Autodesk Fusion 360 part; units mm, degrees
(part 8 of 12)
  arc A873 (-163.0531, -58.1721) -> (-160.5131, -58.1721) centre (-161.7831, -58.1721) ccw
  arc A874 (-124.1631, -55.6321) -> (-126.7031, -55.6321) centre (-125.4331, -55.6321) ccw
  arc A875 (-126.7031, -55.6321) -> (-124.1631, -55.6321) centre (-125.4331, -55.6321) ccw
  arc A876 (-126.7031, -55.6321) -> (-124.1631, -55.6321) centre (-125.4331, -55.6321) ccw
  arc A877 (-124.1631, -55.6321) -> (-126.7031, -55.6321) centre (-125.4331, -55.6321) ccw
  arc A878 (-124.1631, -55.6321) -> (-126.7031, -55.6321) centre (-125.4331, -55.6321) ccw
  arc A879 (-126.7031, -55.6321) -> (-124.1631, -55.6321) centre (-125.4331, -55.6321) ccw
  arc A880 (-130.5131, -58.1721) -> (-133.0531, -58.1721) centre (-131.7831, -58.1721) ccw
  arc A881 (-133.0531, -58.1721) -> (-130.5131, -58.1721) centre (-131.7831, -58.1721) ccw
  arc A882 (-133.0531, -58.1721) -> (-130.5131, -58.1721) centre (-131.7831, -58.1721) ccw
  arc A883 (-130.5131, -58.1721) -> (-133.0531, -58.1721) centre (-131.7831, -58.1721) ccw
  arc A884 (-130.5131, -58.1721) -> (-133.0531, -58.1721) centre (-131.7831, -58.1721) ccw
  arc A885 (-133.0531, -58.1721) -> (-130.5131, -58.1721) centre (-131.7831, -58.1721) ccw
  arc A886 (-94.1631, -55.6321) -> (-96.7031, -55.6321) centre (-95.4331, -55.6321) ccw
  arc A887 (-96.7031, -55.6321) -> (-94.1631, -55.6321) centre (-95.4331, -55.6321) ccw
  arc A888 (-96.7031, -55.6321) -> (-94.1631, -55.6321) centre (-95.4331, -55.6321) ccw
  arc A889 (-94.1631, -55.6321) -> (-96.7031, -55.6321) centre (-95.4331, -55.6321) ccw
  arc A890 (-96.7031, -55.6321) -> (-94.1631, -55.6321) centre (-95.4331, -55.6321) ccw
  arc A891 (-94.1631, -55.6321) -> (-96.7031, -55.6321) centre (-95.4331, -55.6321) ccw
  arc A892 (-103.0531, -58.1721) -> (-100.5131, -58.1721) centre (-101.7831, -58.1721) ccw
  arc A893 (-100.5131, -58.1721) -> (-103.0531, -58.1721) centre (-101.7831, -58.1721) ccw
  arc A894 (-103.0531, -58.1721) -> (-100.5131, -58.1721) centre (-101.7831, -58.1721) ccw
  arc A895 (-100.5131, -58.1721) -> (-103.0531, -58.1721) centre (-101.7831, -58.1721) ccw
  arc A896 (-103.0531, -58.1721) -> (-100.5131, -58.1721) centre (-101.7831, -58.1721) ccw
  arc A897 (-100.5131, -58.1721) -> (-103.0531, -58.1721) centre (-101.7831, -58.1721) ccw
  arc A898 (-66.7031, -55.6321) -> (-64.1631, -55.6321) centre (-65.4331, -55.6321) ccw
  arc A899 (-64.1631, -55.6321) -> (-66.7031, -55.6321) centre (-65.4331, -55.6321) ccw
  arc A900 (-64.1631, -55.6321) -> (-66.7031, -55.6321) centre (-65.4331, -55.6321) ccw
  arc A901 (-66.7031, -55.6321) -> (-64.1631, -55.6321) centre (-65.4331, -55.6321) ccw
  arc A902 (-64.1631, -55.6321) -> (-66.7031, -55.6321) centre (-65.4331, -55.6321) ccw
  arc A903 (-66.7031, -55.6321) -> (-64.1631, -55.6321) centre (-65.4331, -55.6321) ccw
  arc A904 (-70.5131, -58.1721) -> (-73.0531, -58.1721) centre (-71.7831, -58.1721) ccw
  arc A905 (-73.0531, -58.1721) -> (-70.5131, -58.1721) centre (-71.7831, -58.1721) ccw
  arc A906 (-73.0531, -58.1721) -> (-70.5131, -58.1721) centre (-71.7831, -58.1721) ccw
  arc A907 (-70.5131, -58.1721) -> (-73.0531, -58.1721) centre (-71.7831, -58.1721) ccw
  arc A908 (-73.0531, -58.1721) -> (-70.5131, -58.1721) centre (-71.7831, -58.1721) ccw
  arc A909 (-70.5131, -58.1721) -> (-73.0531, -58.1721) centre (-71.7831, -58.1721) ccw
  arc A910 (-34.1631, -55.6321) -> (-36.7031, -55.6321) centre (-35.4331, -55.6321) ccw
  arc A911 (-36.7031, -55.6321) -> (-34.1631, -55.6321) centre (-35.4331, -55.6321) ccw
  arc A912 (-34.1631, -55.6321) -> (-36.7031, -55.6321) centre (-35.4331, -55.6321) ccw
  arc A913 (-36.7031, -55.6321) -> (-34.1631, -55.6321) centre (-35.4331, -55.6321) ccw
  arc A914 (-34.1631, -55.6321) -> (-36.7031, -55.6321) centre (-35.4331, -55.6321) ccw
  arc A915 (-36.7031, -55.6321) -> (-34.1631, -55.6321) centre (-35.4331, -55.6321) ccw
  arc A916 (-43.0531, -58.1721) -> (-40.5131, -58.1721) centre (-41.7831, -58.1721) ccw
  arc A917 (-40.5131, -58.1721) -> (-43.0531, -58.1721) centre (-41.7831, -58.1721) ccw
  arc A918 (-40.5131, -58.1721) -> (-43.0531, -58.1721) centre (-41.7831, -58.1721) ccw
  arc A919 (-43.0531, -58.1721) -> (-40.5131, -58.1721) centre (-41.7831, -58.1721) ccw
  arc A920 (-43.0531, -58.1721) -> (-40.5131, -58.1721) centre (-41.7831, -58.1721) ccw
  arc A921 (-40.5131, -58.1721) -> (-43.0531, -58.1721) centre (-41.7831, -58.1721) ccw
  arc A922 (8.763, -56.6421) -> (6.223, -56.6421) centre (7.493, -56.6421) ccw
  arc A923 (6.223, -56.6421) -> (8.763, -56.6421) centre (7.493, -56.6421) ccw
  arc A924 (6.223, -56.6421) -> (8.763, -56.6421) centre (7.493, -56.6421) ccw
  arc A925 (8.763, -56.6421) -> (6.223, -56.6421) centre (7.493, -56.6421) ccw
  arc A926 (6.223, -56.6421) -> (8.763, -56.6421) centre (7.493, -56.6421) ccw
  arc A927 (8.763, -56.6421) -> (6.223, -56.6421) centre (7.493, -56.6421) ccw
  arc A928 (2.413, -59.1821) -> (-0.127, -59.1821) centre (1.143, -59.1821) ccw
  arc A929 (-0.127, -59.1821) -> (2.413, -59.1821) centre (1.143, -59.1821) ccw
  arc A930 (-0.127, -59.1821) -> (2.413, -59.1821) centre (1.143, -59.1821) ccw
  arc A931 (2.413, -59.1821) -> (-0.127, -59.1821) centre (1.143, -59.1821) ccw
  arc A932 (-0.127, -59.1821) -> (2.413, -59.1821) centre (1.143, -59.1821) ccw
  arc A933 (2.413, -59.1821) -> (-0.127, -59.1821) centre (1.143, -59.1821) ccw
  arc A934 (-175.4509, -86.7412) -> (-172.9108, -86.7412) centre (-174.1808, -86.7412) ccw
  arc A935 (-172.9108, -86.7412) -> (-175.4509, -86.7412) centre (-174.1808, -86.7412) ccw
  arc A936 (-175.4509, -86.7412) -> (-172.9108, -86.7412) centre (-174.1808, -86.7412) ccw
  arc A937 (-172.9108, -86.7412) -> (-175.4509, -86.7412) centre (-174.1808, -86.7412) ccw
  arc A938 (-172.9108, -86.7412) -> (-175.4509, -86.7412) centre (-174.1808, -86.7412) ccw
  arc A939 (-175.4509, -86.7412) -> (-172.9108, -86.7412) centre (-174.1808, -86.7412) ccw
  arc A940 (-181.8009, -89.2812) -> (-179.2609, -89.2812) centre (-180.5309, -89.2812) ccw
  arc A941 (-179.2609, -89.2812) -> (-181.8009, -89.2812) centre (-180.5309, -89.2812) ccw
  arc A942 (-181.8009, -89.2812) -> (-179.2609, -89.2812) centre (-180.5309, -89.2812) ccw
  arc A943 (-179.2609, -89.2812) -> (-181.8009, -89.2812) centre (-180.5309, -89.2812) ccw
  arc A944 (-181.8009, -89.2812) -> (-179.2609, -89.2812) centre (-180.5309, -89.2812) ccw
  arc A945 (-179.2609, -89.2812) -> (-181.8009, -89.2812) centre (-180.5309, -89.2812) ccw
  arc A946 (57.6581, -64.0081) -> (55.1181, -64.0081) centre (56.3881, -64.0081) ccw
  arc A947 (55.1181, -64.0081) -> (57.6581, -64.0081) centre (56.3881, -64.0081) ccw
  arc A948 (55.1181, -64.0081) -> (57.6581, -64.0081) centre (56.3881, -64.0081) ccw
  arc A949 (57.6581, -64.0081) -> (55.1181, -64.0081) centre (56.3881, -64.0081) ccw
  arc A950 (55.1181, -64.0081) -> (57.6581, -64.0081) centre (56.3881, -64.0081) ccw
  arc A951 (57.6581, -64.0081) -> (55.1181, -64.0081) centre (56.3881, -64.0081) ccw
  arc A952 (48.7681, -66.5481) -> (51.3081, -66.5481) centre (50.0381, -66.5481) ccw
  arc A953 (51.3081, -66.5481) -> (48.7681, -66.5481) centre (50.0381, -66.5481) ccw
  arc A954 (48.7681, -66.5481) -> (51.3081, -66.5481) centre (50.0381, -66.5481) ccw
  arc A955 (51.3081, -66.5481) -> (48.7681, -66.5481) centre (50.0381, -66.5481) ccw
  arc A956 (51.3081, -66.5481) -> (48.7681, -66.5481) centre (50.0381, -66.5481) ccw
  arc A957 (48.7681, -66.5481) -> (51.3081, -66.5481) centre (50.0381, -66.5481) ccw
  arc A958 (-142.4943, -86.7412) -> (-145.0343, -86.7412) centre (-143.7643, -86.7412) ccw
  arc A959 (-145.0343, -86.7412) -> (-142.4943, -86.7412) centre (-143.7643, -86.7412) ccw
  arc A960 (-145.0343, -86.7412) -> (-142.4943, -86.7412) centre (-143.7643, -86.7412) ccw
  arc A961 (-142.4943, -86.7412) -> (-145.0343, -86.7412) centre (-143.7643, -86.7412) ccw
  arc A962 (-145.0343, -86.7412) -> (-142.4943, -86.7412) centre (-143.7643, -86.7412) ccw
  arc A963 (-142.4943, -86.7412) -> (-145.0343, -86.7412) centre (-143.7643, -86.7412) ccw
  arc A964 (-151.3844, -89.2812) -> (-148.8443, -89.2812) centre (-150.1144, -89.2812) ccw
  arc A965 (-148.8443, -89.2812) -> (-151.3844, -89.2812) centre (-150.1144, -89.2812) ccw
  arc A966 (-148.8443, -89.2812) -> (-151.3844, -89.2812) centre (-150.1144, -89.2812) ccw
  arc A967 (-151.3844, -89.2812) -> (-148.8443, -89.2812) centre (-150.1144, -89.2812) ccw
  arc A968 (-148.8443, -89.2812) -> (-151.3844, -89.2812) centre (-150.1144, -89.2812) ccw
  arc A969 (-151.3844, -89.2812) -> (-148.8443, -89.2812) centre (-150.1144, -89.2812) ccw
  arc A970 (-112.0778, -86.7412) -> (-114.6178, -86.7412) centre (-113.3478, -86.7412) ccw
  arc A971 (-114.6178, -86.7412) -> (-112.0778, -86.7412) centre (-113.3478, -86.7412) ccw
  arc A972 (-112.0778, -86.7412) -> (-114.6178, -86.7412) centre (-113.3478, -86.7412) ccw
  arc A973 (-114.6178, -86.7412) -> (-112.0778, -86.7412) centre (-113.3478, -86.7412) ccw
  arc A974 (-114.6178, -86.7412) -> (-112.0778, -86.7412) centre (-113.3478, -86.7412) ccw
  arc A975 (-112.0778, -86.7412) -> (-114.6178, -86.7412) centre (-113.3478, -86.7412) ccw
  arc A976 (-118.4278, -89.2812) -> (-120.9678, -89.2812) centre (-119.6978, -89.2812) ccw
  arc A977 (-120.9678, -89.2812) -> (-118.4278, -89.2812) centre (-119.6978, -89.2812) ccw
  arc A978 (-118.4278, -89.2812) -> (-120.9678, -89.2812) centre (-119.6978, -89.2812) ccw
  arc A979 (-120.9678, -89.2812) -> (-118.4278, -89.2812) centre (-119.6978, -89.2812) ccw
  arc A980 (-118.4278, -89.2812) -> (-120.9678, -89.2812) centre (-119.6978, -89.2812) ccw
  arc A981 (-120.9678, -89.2812) -> (-118.4278, -89.2812) centre (-119.6978, -89.2812) ccw
  arc A982 (-84.2012, -86.7412) -> (-81.6612, -86.7412) centre (-82.9312, -86.7412) ccw
  arc A983 (-81.6612, -86.7412) -> (-84.2012, -86.7412) centre (-82.9312, -86.7412) ccw
  arc A984 (-84.2012, -86.7412) -> (-81.6612, -86.7412) centre (-82.9312, -86.7412) ccw
  arc A985 (-81.6612, -86.7412) -> (-84.2012, -86.7412) centre (-82.9312, -86.7412) ccw
  arc A986 (-81.6612, -86.7412) -> (-84.2012, -86.7412) centre (-82.9312, -86.7412) ccw
  arc A987 (-84.2012, -86.7412) -> (-81.6612, -86.7412) centre (-82.9312, -86.7412) ccw
  arc A988 (-88.0112, -89.2812) -> (-90.5512, -89.2812) centre (-89.2812, -89.2812) ccw
  arc A989 (-90.5512, -89.2812) -> (-88.0112, -89.2812) centre (-89.2812, -89.2812) ccw
  arc A990 (-90.5512, -89.2812) -> (-88.0112, -89.2812) centre (-89.2812, -89.2812) ccw
  arc A991 (-88.0112, -89.2812) -> (-90.5512, -89.2812) centre (-89.2812, -89.2812) ccw
  arc A992 (-88.0112, -89.2812) -> (-90.5512, -89.2812) centre (-89.2812, -89.2812) ccw
  arc A993 (-90.5512, -89.2812) -> (-88.0112, -89.2812) centre (-89.2812, -89.2812) ccw
  arc A994 (-51.2446, -86.7412) -> (-53.7846, -86.7412) centre (-52.5146, -86.7412) ccw
  arc A995 (-53.7846, -86.7412) -> (-51.2446, -86.7412) centre (-52.5146, -86.7412) ccw
  arc A996 (-51.2446, -86.7412) -> (-53.7846, -86.7412) centre (-52.5146, -86.7412) ccw
  arc A997 (-53.7846, -86.7412) -> (-51.2446, -86.7412) centre (-52.5146, -86.7412) ccw
  arc A998 (-53.7846, -86.7412) -> (-51.2446, -86.7412) centre (-52.5146, -86.7412) ccw
  arc A999 (-51.2446, -86.7412) -> (-53.7846, -86.7412) centre (-52.5146, -86.7412) ccw
  arc A1000 (-60.1346, -89.2812) -> (-57.5946, -89.2812) centre (-58.8646, -89.2812) ccw
  arc A1001 (-57.5946, -89.2812) -> (-60.1346, -89.2812) centre (-58.8646, -89.2812) ccw
  arc A1002 (-60.1346, -89.2812) -> (-57.5946, -89.2812) centre (-58.8646, -89.2812) ccw
  arc A1003 (-57.5946, -89.2812) -> (-60.1346, -89.2812) centre (-58.8646, -89.2812) ccw
  arc A1004 (-57.5946, -89.2812) -> (-60.1346, -89.2812) centre (-58.8646, -89.2812) ccw
  arc A1005 (-60.1346, -89.2812) -> (-57.5946, -89.2812) centre (-58.8646, -89.2812) ccw
  arc A1006 (-20.828, -86.7412) -> (-23.368, -86.7412) centre (-22.098, -86.7412) ccw
  arc A1007 (-23.368, -86.7412) -> (-20.828, -86.7412) centre (-22.098, -86.7412) ccw
  arc A1008 (-20.828, -86.7412) -> (-23.368, -86.7412) centre (-22.098, -86.7412) ccw
  arc A1009 (-23.368, -86.7412) -> (-20.828, -86.7412) centre (-22.098, -86.7412) ccw
  arc A1010 (-20.828, -86.7412) -> (-23.368, -86.7412) centre (-22.098, -86.7412) ccw
  arc A1011 (-23.368, -86.7412) -> (-20.828, -86.7412) centre (-22.098, -86.7412) ccw
  arc A1012 (-29.7181, -89.2812) -> (-27.1781, -89.2812) centre (-28.4481, -89.2812) ccw
  arc A1013 (-27.1781, -89.2812) -> (-29.7181, -89.2812) centre (-28.4481, -89.2812) ccw
  arc A1014 (-29.7181, -89.2812) -> (-27.1781, -89.2812) centre (-28.4481, -89.2812) ccw
  arc A1015 (-27.1781, -89.2812) -> (-29.7181, -89.2812) centre (-28.4481, -89.2812) ccw
  arc A1016 (-29.7181, -89.2812) -> (-27.1781, -89.2812) centre (-28.4481, -89.2812) ccw
  arc A1017 (-27.1781, -89.2812) -> (-29.7181, -89.2812) centre (-28.4481, -89.2812) ccw
  arc A1018 (9.525, -86.8424) -> (6.985, -86.8424) centre (8.255, -86.8424) ccw
  arc A1019 (6.985, -86.8424) -> (9.525, -86.8424) centre (8.255, -86.8424) ccw
  arc A1020 (9.525, -86.8424) -> (6.985, -86.8424) centre (8.255, -86.8424) ccw
  arc A1021 (6.985, -86.8424) -> (9.525, -86.8424) centre (8.255, -86.8424) ccw
  arc A1022 (9.525, -86.8424) -> (6.985, -86.8424) centre (8.255, -86.8424) ccw
  arc A1023 (6.985, -86.8424) -> (9.525, -86.8424) centre (8.255, -86.8424) ccw
  arc A1024 (0.635, -89.3824) -> (3.175, -89.3824) centre (1.905, -89.3824) ccw
  arc A1025 (3.175, -89.3824) -> (0.635, -89.3824) centre (1.905, -89.3824) ccw
  arc A1026 (0.635, -89.3824) -> (3.175, -89.3824) centre (1.905, -89.3824) ccw
  arc A1027 (3.175, -89.3824) -> (0.635, -89.3824) centre (1.905, -89.3824) ccw
  arc A1028 (0.635, -89.3824) -> (3.175, -89.3824) centre (1.905, -89.3824) ccw
  arc A1029 (3.175, -89.3824) -> (0.635, -89.3824) centre (1.905, -89.3824) ccw
  arc A1030 (35.1911, -82.8042) -> (36.6911, -82.8042) centre (35.9411, -82.8042) ccw
  arc A1031 (36.6911, -82.8042) -> (35.1911, -82.8042) centre (35.9411, -82.8042) ccw
  arc A1032 (35.1911, -82.8042) -> (36.6911, -82.8042) centre (35.9411, -82.8042) ccw
  arc A1033 (36.6911, -82.8042) -> (35.1911, -82.8042) centre (35.9411, -82.8042) ccw
  arc A1034 (36.6911, -82.8042) -> (35.1911, -82.8042) centre (35.9411, -82.8042) ccw
  arc A1035 (35.1911, -82.8042) -> (36.6911, -82.8042) centre (35.9411, -82.8042) ccw
  arc A1036 (35.1911, -80.2642) -> (36.6911, -80.2642) centre (35.9411, -80.2642) ccw
  arc A1037 (36.6911, -80.2642) -> (35.1911, -80.2642) centre (35.9411, -80.2642) ccw
  arc A1038 (35.1911, -80.2642) -> (36.6911, -80.2642) centre (35.9411, -80.2642) ccw
  arc A1039 (36.6911, -80.2642) -> (35.1911, -80.2642) centre (35.9411, -80.2642) ccw
  arc A1040 (35.1911, -80.2642) -> (36.6911, -80.2642) centre (35.9411, -80.2642) ccw
  arc A1041 (36.6911, -80.2642) -> (35.1911, -80.2642) centre (35.9411, -80.2642) ccw
  arc A1042 (36.6911, -77.7242) -> (35.1911, -77.7242) centre (35.9411, -77.7242) ccw
  arc A1043 (35.1911, -77.7242) -> (36.6911, -77.7242) centre (35.9411, -77.7242) ccw
  arc A1044 (36.6911, -77.7242) -> (35.1911, -77.7242) centre (35.9411, -77.7242) ccw
  arc A1045 (35.1911, -77.7242) -> (36.6911, -77.7242) centre (35.9411, -77.7242) ccw
  arc A1046 (36.6911, -77.7242) -> (35.1911, -77.7242) centre (35.9411, -77.7242) ccw
  arc A1047 (35.1911, -77.7242) -> (36.6911, -77.7242) centre (35.9411, -77.7242) ccw
  arc A1048 (36.6911, -75.1842) -> (35.1911, -75.1842) centre (35.9411, -75.1842) ccw
  arc A1049 (35.1911, -75.1842) -> (36.6911, -75.1842) centre (35.9411, -75.1842) ccw
  arc A1050 (36.6911, -75.1842) -> (35.1911, -75.1842) centre (35.9411, -75.1842) ccw
  arc A1051 (35.1911, -75.1842) -> (36.6911, -75.1842) centre (35.9411, -75.1842) ccw
  arc A1052 (36.6911, -75.1842) -> (35.1911, -75.1842) centre (35.9411, -75.1842) ccw
  arc A1053 (35.1911, -75.1842) -> (36.6911, -75.1842) centre (35.9411, -75.1842) ccw
  arc A1054 (36.6911, -72.6441) -> (35.1911, -72.6441) centre (35.9411, -72.6441) ccw
  arc A1055 (35.1911, -72.6441) -> (36.6911, -72.6441) centre (35.9411, -72.6441) ccw
  arc A1056 (35.1911, -72.6441) -> (36.6911, -72.6441) centre (35.9411, -72.6441) ccw
  arc A1057 (36.6911, -72.6441) -> (35.1911, -72.6441) centre (35.9411, -72.6441) ccw
  arc A1058 (36.6911, -72.6441) -> (35.1911, -72.6441) centre (35.9411, -72.6441) ccw
  arc A1059 (35.1911, -72.6441) -> (36.6911, -72.6441) centre (35.9411, -72.6441) ccw
  arc A1060 (36.6911, -70.1041) -> (35.1911, -70.1041) centre (35.9411, -70.1041) ccw
  arc A1061 (35.1911, -70.1041) -> (36.6911, -70.1041) centre (35.9411, -70.1041) ccw
  arc A1062 (36.6911, -70.1041) -> (35.1911, -70.1041) centre (35.9411, -70.1041) ccw
  arc A1063 (35.1911, -70.1041) -> (36.6911, -70.1041) centre (35.9411, -70.1041) ccw
  arc A1064 (36.6911, -70.1041) -> (35.1911, -70.1041) centre (35.9411, -70.1041) ccw
  arc A1065 (35.1911, -70.1041) -> (36.6911, -70.1041) centre (35.9411, -70.1041) ccw
  arc A1066 (36.6911, -67.5641) -> (35.1911, -67.5641) centre (35.9411, -67.5641) ccw
  arc A1067 (35.1911, -67.5641) -> (36.6911, -67.5641) centre (35.9411, -67.5641) ccw
  arc A1068 (36.6911, -67.5641) -> (35.1911, -67.5641) centre (35.9411, -67.5641) ccw
  arc A1069 (35.1911, -67.5641) -> (36.6911, -67.5641) centre (35.9411, -67.5641) ccw
  arc A1070 (36.6911, -67.5641) -> (35.1911, -67.5641) centre (35.9411, -67.5641) ccw
  arc A1071 (35.1911, -67.5641) -> (36.6911, -67.5641) centre (35.9411, -67.5641) ccw
  arc A1072 (35.1911, -65.0241) -> (36.6911, -65.0241) centre (35.9411, -65.0241) ccw
  arc A1073 (36.6911, -65.0241) -> (35.1911, -65.0241) centre (35.9411, -65.0241) ccw
  arc A1074 (36.6911, -65.0241) -> (35.1911, -65.0241) centre (35.9411, -65.0241) ccw
  arc A1075 (35.1911, -65.0241) -> (36.6911, -65.0241) centre (35.9411, -65.0241) ccw
  arc A1076 (35.1911, -65.0241) -> (36.6911, -65.0241) centre (35.9411, -65.0241) ccw
  arc A1077 (36.6911, -65.0241) -> (35.1911, -65.0241) centre (35.9411, -65.0241) ccw
  arc A1078 (36.6911, -62.4841) -> (35.1911, -62.4841) centre (35.9411, -62.4841) ccw
  arc A1079 (35.1911, -62.4841) -> (36.6911, -62.4841) centre (35.9411, -62.4841) ccw
  arc A1080 (36.6911, -62.4841) -> (35.1911, -62.4841) centre (35.9411, -62.4841) ccw
  arc A1081 (35.1911, -62.4841) -> (36.6911, -62.4841) centre (35.9411, -62.4841) ccw
  arc A1082 (35.1911, -62.4841) -> (36.6911, -62.4841) centre (35.9411, -62.4841) ccw
  arc A1083 (36.6911, -62.4841) -> (35.1911, -62.4841) centre (35.9411, -62.4841) ccw
  arc A1084 (35.1911, -59.9441) -> (36.6911, -59.9441) centre (35.9411, -59.9441) ccw
  arc A1085 (36.6911, -59.9441) -> (35.1911, -59.9441) centre (35.9411, -59.9441) ccw
  arc A1086 (36.6911, -59.9441) -> (35.1911, -59.9441) centre (35.9411, -59.9441) ccw
  arc A1087 (35.1911, -59.9441) -> (36.6911, -59.9441) centre (35.9411, -59.9441) ccw
  arc A1088 (35.1911, -59.9441) -> (36.6911, -59.9441) centre (35.9411, -59.9441) ccw
  arc A1089 (36.6911, -59.9441) -> (35.1911, -59.9441) centre (35.9411, -59.9441) ccw
  arc A1090 (35.1911, -57.4041) -> (36.6911, -57.4041) centre (35.9411, -57.4041) ccw
  arc A1091 (36.6911, -57.4041) -> (35.1911, -57.4041) centre (35.9411, -57.4041) ccw
  arc A1092 (35.1911, -57.4041) -> (36.6911, -57.4041) centre (35.9411, -57.4041) ccw
  arc A1093 (36.6911, -57.4041) -> (35.1911, -57.4041) centre (35.9411, -57.4041) ccw
  arc A1094 (36.6911, -57.4041) -> (35.1911, -57.4041) centre (35.9411, -57.4041) ccw
  arc A1095 (35.1911, -57.4041) -> (36.6911, -57.4041) centre (35.9411, -57.4041) ccw
  arc A1096 (36.6911, -54.8641) -> (35.1911, -54.8641) centre (35.9411, -54.8641) ccw
  arc A1097 (35.1911, -54.8641) -> (36.6911, -54.8641) centre (35.9411, -54.8641) ccw
  arc A1098 (36.6911, -54.8641) -> (35.1911, -54.8641) centre (35.9411, -54.8641) ccw
  arc A1099 (35.1911, -54.8641) -> (36.6911, -54.8641) centre (35.9411, -54.8641) ccw
  arc A1100 (35.1911, -54.8641) -> (36.6911, -54.8641) centre (35.9411, -54.8641) ccw
  arc A1101 (36.6911, -54.8641) -> (35.1911, -54.8641) centre (35.9411, -54.8641) ccw
  arc A1102 (36.6911, -52.3241) -> (35.1911, -52.3241) centre (35.9411, -52.3241) ccw
  arc A1103 (35.1911, -52.3241) -> (36.6911, -52.3241) centre (35.9411, -52.3241) ccw
  arc A1104 (35.1911, -52.3241) -> (36.6911, -52.3241) centre (35.9411, -52.3241) ccw
  arc A1105 (36.6911, -52.3241) -> (35.1911, -52.3241) centre (35.9411, -52.3241) ccw
  arc A1106 (36.6911, -52.3241) -> (35.1911, -52.3241) centre (35.9411, -52.3241) ccw
  arc A1107 (35.1911, -52.3241) -> (36.6911, -52.3241) centre (35.9411, -52.3241) ccw
  arc A1108 (35.1911, -49.7841) -> (36.6911, -49.7841) centre (35.9411, -49.7841) ccw
  arc A1109 (36.6911, -49.7841) -> (35.1911, -49.7841) centre (35.9411, -49.7841) ccw
  arc A1110 (35.1911, -49.7841) -> (36.6911, -49.7841) centre (35.9411, -49.7841) ccw
  arc A1111 (36.6911, -49.7841) -> (35.1911, -49.7841) centre (35.9411, -49.7841) ccw
  arc A1112 (35.1911, -49.7841) -> (36.6911, -49.7841) centre (35.9411, -49.7841) ccw
  arc A1113 (36.6911, -49.7841) -> (35.1911, -49.7841) centre (35.9411, -49.7841) ccw
  arc A1114 (29.0711, -82.8042) -> (27.5711, -82.8042) centre (28.3211, -82.8042) ccw
  arc A1115 (27.5711, -82.8042) -> (29.0711, -82.8042) centre (28.3211, -82.8042) ccw
  arc A1116 (29.0711, -82.8042) -> (27.5711, -82.8042) centre (28.3211, -82.8042) ccw
  arc A1117 (27.5711, -82.8042) -> (29.0711, -82.8042) centre (28.3211, -82.8042) ccw
  arc A1118 (27.5711, -82.8042) -> (29.0711, -82.8042) centre (28.3211, -82.8042) ccw
  arc A1119 (29.0711, -82.8042) -> (27.5711, -82.8042) centre (28.3211, -82.8042) ccw
  arc A1120 (27.5711, -80.2642) -> (29.0711, -80.2642) centre (28.3211, -80.2642) ccw
  arc A1121 (29.0711, -80.2642) -> (27.5711, -80.2642) centre (28.3211, -80.2642) ccw
  arc A1122 (27.5711, -80.2642) -> (29.0711, -80.2642) centre (28.3211, -80.2642) ccw
  arc A1123 (29.0711, -80.2642) -> (27.5711, -80.2642) centre (28.3211, -80.2642) ccw
  arc A1124 (29.0711, -80.2642) -> (27.5711, -80.2642) centre (28.3211, -80.2642) ccw
  arc A1125 (27.5711, -80.2642) -> (29.0711, -80.2642) centre (28.3211, -80.2642) ccw
  arc A1126 (27.5711, -77.7242) -> (29.0711, -77.7242) centre (28.3211, -77.7242) ccw
  arc A1127 (29.0711, -77.7242) -> (27.5711, -77.7242) centre (28.3211, -77.7242) ccw
  arc A1128 (29.0711, -77.7242) -> (27.5711, -77.7242) centre (28.3211, -77.7242) ccw
  arc A1129 (27.5711, -77.7242) -> (29.0711, -77.7242) centre (28.3211, -77.7242) ccw
  arc A1130 (27.5711, -77.7242) -> (29.0711, -77.7242) centre (28.3211, -77.7242) ccw
  arc A1131 (29.0711, -77.7242) -> (27.5711, -77.7242) centre (28.3211, -77.7242) ccw
  arc A1132 (29.0711, -75.1842) -> (27.5711, -75.1842) centre (28.3211, -75.1842) ccw
  arc A1133 (27.5711, -75.1842) -> (29.0711, -75.1842) centre (28.3211, -75.1842) ccw
  arc A1134 (27.5711, -75.1842) -> (29.0711, -75.1842) centre (28.3211, -75.1842) ccw
  arc A1135 (29.0711, -75.1842) -> (27.5711, -75.1842) centre (28.3211, -75.1842) ccw
  arc A1136 (27.5711, -75.1842) -> (29.0711, -75.1842) centre (28.3211, -75.1842) ccw
  arc A1137 (29.0711, -75.1842) -> (27.5711, -75.1842) centre (28.3211, -75.1842) ccw
  arc A1138 (27.5711, -72.6441) -> (29.0711, -72.6441) centre (28.3211, -72.6441) ccw
  arc A1139 (29.0711, -72.6441) -> (27.5711, -72.6441) centre (28.3211, -72.6441) ccw
  arc A1140 (29.0711, -72.6441) -> (27.5711, -72.6441) centre (28.3211, -72.6441) ccw
  arc A1141 (27.5711, -72.6441) -> (29.0711, -72.6441) centre (28.3211, -72.6441) ccw
  arc A1142 (29.0711, -72.6441) -> (27.5711, -72.6441) centre (28.3211, -72.6441) ccw
  arc A1143 (27.5711, -72.6441) -> (29.0711, -72.6441) centre (28.3211, -72.6441) ccw
  arc A1144 (27.5711, -70.1041) -> (29.0711, -70.1041) centre (28.3211, -70.1041) ccw
  arc A1145 (29.0711, -70.1041) -> (27.5711, -70.1041) centre (28.3211, -70.1041) ccw
  arc A1146 (27.5711, -70.1041) -> (29.0711, -70.1041) centre (28.3211, -70.1041) ccw
  arc A1147 (29.0711, -70.1041) -> (27.5711, -70.1041) centre (28.3211, -70.1041) ccw
  arc A1148 (27.5711, -70.1041) -> (29.0711, -70.1041) centre (28.3211, -70.1041) ccw
  arc A1149 (29.0711, -70.1041) -> (27.5711, -70.1041) centre (28.3211, -70.1041) ccw
  arc A1150 (27.5711, -67.5641) -> (29.0711, -67.5641) centre (28.3211, -67.5641) ccw
  arc A1151 (29.0711, -67.5641) -> (27.5711, -67.5641) centre (28.3211, -67.5641) ccw
  arc A1152 (29.0711, -67.5641) -> (27.5711, -67.5641) centre (28.3211, -67.5641) ccw
  arc A1153 (27.5711, -67.5641) -> (29.0711, -67.5641) centre (28.3211, -67.5641) ccw
  arc A1154 (27.5711, -67.5641) -> (29.0711, -67.5641) centre (28.3211, -67.5641) ccw
  arc A1155 (29.0711, -67.5641) -> (27.5711, -67.5641) centre (28.3211, -67.5641) ccw
  arc A1156 (27.5711, -65.0241) -> (29.0711, -65.0241) centre (28.3211, -65.0241) ccw
  arc A1157 (29.0711, -65.0241) -> (27.5711, -65.0241) centre (28.3211, -65.0241) ccw
  arc A1158 (29.0711, -65.0241) -> (27.5711, -65.0241) centre (28.3211, -65.0241) ccw
  arc A1159 (27.5711, -65.0241) -> (29.0711, -65.0241) centre (28.3211, -65.0241) ccw
  arc A1160 (27.5711, -65.0241) -> (29.0711, -65.0241) centre (28.3211, -65.0241) ccw
  arc A1161 (29.0711, -65.0241) -> (27.5711, -65.0241) centre (28.3211, -65.0241) ccw
  arc A1162 (27.5711, -62.4841) -> (29.0711, -62.4841) centre (28.3211, -62.4841) ccw
  arc A1163 (29.0711, -62.4841) -> (27.5711, -62.4841) centre (28.3211, -62.4841) ccw
  arc A1164 (27.5711, -62.4841) -> (29.0711, -62.4841) centre (28.3211, -62.4841) ccw
  arc A1165 (29.0711, -62.4841) -> (27.5711, -62.4841) centre (28.3211, -62.4841) ccw
  arc A1166 (29.0711, -62.4841) -> (27.5711, -62.4841) centre (28.3211, -62.4841) ccw
  arc A1167 (27.5711, -62.4841) -> (29.0711, -62.4841) centre (28.3211, -62.4841) ccw
  arc A1168 (29.0711, -59.9441) -> (27.5711, -59.9441) centre (28.3211, -59.9441) ccw
  arc A1169 (27.5711, -59.9441) -> (29.0711, -59.9441) centre (28.3211, -59.9441) ccw
  arc A1170 (29.0711, -59.9441) -> (27.5711, -59.9441) centre (28.3211, -59.9441) ccw
  arc A1171 (27.5711, -59.9441) -> (29.0711, -59.9441) centre (28.3211, -59.9441) ccw
  arc A1172 (29.0711, -59.9441) -> (27.5711, -59.9441) centre (28.3211, -59.9441) ccw
  arc A1173 (27.5711, -59.9441) -> (29.0711, -59.9441) centre (28.3211, -59.9441) ccw
  arc A1174 (27.5711, -57.4041) -> (29.0711, -57.4041) centre (28.3211, -57.4041) ccw
  arc A1175 (29.0711, -57.4041) -> (27.5711, -57.4041) centre (28.3211, -57.4041) ccw
  arc A1176 (29.0711, -57.4041) -> (27.5711, -57.4041) centre (28.3211, -57.4041) ccw
  arc A1177 (27.5711, -57.4041) -> (29.0711, -57.4041) centre (28.3211, -57.4041) ccw
  arc A1178 (27.5711, -57.4041) -> (29.0711, -57.4041) centre (28.3211, -57.4041) ccw
  arc A1179 (29.0711, -57.4041) -> (27.5711, -57.4041) centre (28.3211, -57.4041) ccw
  arc A1180 (29.0711, -54.8641) -> (27.5711, -54.8641) centre (28.3211, -54.8641) ccw
  arc A1181 (27.5711, -54.8641) -> (29.0711, -54.8641) centre (28.3211, -54.8641) ccw
  arc A1182 (29.0711, -54.8641) -> (27.5711, -54.8641) centre (28.3211, -54.8641) ccw
  arc A1183 (27.5711, -54.8641) -> (29.0711, -54.8641) centre (28.3211, -54.8641) ccw
  arc A1184 (29.0711, -54.8641) -> (27.5711, -54.8641) centre (28.3211, -54.8641) ccw
  arc A1185 (27.5711, -54.8641) -> (29.0711, -54.8641) centre (28.3211, -54.8641) ccw
  arc A1186 (29.0711, -52.3241) -> (27.5711, -52.3241) centre (28.3211, -52.3241) ccw
  arc A1187 (27.5711, -52.3241) -> (29.0711, -52.3241) centre (28.3211, -52.3241) ccw
  arc A1188 (27.5711, -52.3241) -> (29.0711, -52.3241) centre (28.3211, -52.3241) ccw
  arc A1189 (29.0711, -52.3241) -> (27.5711, -52.3241) centre (28.3211, -52.3241) ccw
  arc A1190 (27.5711, -52.3241) -> (29.0711, -52.3241) centre (28.3211, -52.3241) ccw
  arc A1191 (29.0711, -52.3241) -> (27.5711, -52.3241) centre (28.3211, -52.3241) ccw
  line L232 (27.5711, -49.0341) -> (29.0711, -49.0341)
  line L233 (29.0711, -50.5341) -> (27.5711, -50.5341)
  line L234 (27.5711, -50.5341) -> (27.5711, -49.0341)
  line L235 (29.0711, -49.0341) -> (29.0711, -50.5341)
  line L236 (29.0711, -49.0341) -> (29.0711, -50.5341)
  line L237 (29.0711, -50.5341) -> (27.5711, -50.5341)
  line L238 (27.5711, -50.5341) -> (27.5711, -49.0341)
  line L239 (27.5711, -49.0341) -> (29.0711, -49.0341)
  line L240 (27.5711, -49.0341) -> (29.0711, -49.0341)
  line L241 (29.0711, -49.0341) -> (29.0711, -50.5341)
  line L242 (27.5711, -50.5341) -> (27.5711, -49.0341)
  line L243 (29.0711, -50.5341) -> (27.5711, -50.5341)
  arc A1192 (79.1332, -69.0881) -> (80.6332, -69.0881) centre (79.8832, -69.0881) ccw
  arc A1193 (80.6332, -69.0881) -> (79.1332, -69.0881) centre (79.8832, -69.0881) ccw
  arc A1194 (80.6332, -69.0881) -> (79.1332, -69.0881) centre (79.8832, -69.0881) ccw
  arc A1195 (79.1332, -69.0881) -> (80.6332, -69.0881) centre (79.8832, -69.0881) ccw
  arc A1196 (80.6332, -69.0881) -> (79.1332, -69.0881) centre (79.8832, -69.0881) ccw
  arc A1197 (79.1332, -69.0881) -> (80.6332, -69.0881) centre (79.8832, -69.0881) ccw
  arc A1198 (80.6332, -66.5481) -> (79.1332, -66.5481) centre (79.8832, -66.5481) ccw
  arc A1199 (79.1332, -66.5481) -> (80.6332, -66.5481) centre (79.8832, -66.5481) ccw
  arc A1200 (79.1332, -66.5481) -> (80.6332, -66.5481) centre (79.8832, -66.5481) ccw
  arc A1201 (80.6332, -66.5481) -> (79.1332, -66.5481) centre (79.8832, -66.5481) ccw
  arc A1202 (79.1332, -66.5481) -> (80.6332, -66.5481) centre (79.8832, -66.5481) ccw
  arc A1203 (80.6332, -66.5481) -> (79.1332, -66.5481) centre (79.8832, -66.5481) ccw
  arc A1204 (79.1332, -64.0081) -> (80.6332, -64.0081) centre (79.8832, -64.0081) ccw
  arc A1205 (80.6332, -64.0081) -> (79.1332, -64.0081) centre (79.8832, -64.0081) ccw
  arc A1206 (79.1332, -64.0081) -> (80.6332, -64.0081) centre (79.8832, -64.0081) ccw
  arc A1207 (80.6332, -64.0081) -> (79.1332, -64.0081) centre (79.8832, -64.0081) ccw
  arc A1208 (79.1332, -64.0081) -> (80.6332, -64.0081) centre (79.8832, -64.0081) ccw
  arc A1209 (80.6332, -64.0081) -> (79.1332, -64.0081) centre (79.8832, -64.0081) ccw
  arc A1210 (79.1332, -61.4681) -> (80.6332, -61.4681) centre (79.8832, -61.4681) ccw
  arc A1211 (80.6332, -61.4681) -> (79.1332, -61.4681) centre (79.8832, -61.4681) ccw
  arc A1212 (79.1332, -61.4681) -> (80.6332, -61.4681) centre (79.8832, -61.4681) ccw
  arc A1213 (80.6332, -61.4681) -> (79.1332, -61.4681) centre (79.8832, -61.4681) ccw
  arc A1214 (80.6332, -61.4681) -> (79.1332, -61.4681) centre (79.8832, -61.4681) ccw
  arc A1215 (79.1332, -61.4681) -> (80.6332, -61.4681) centre (79.8832, -61.4681) ccw
  arc A1216 (79.1332, -58.9281) -> (80.6332, -58.9281) centre (79.8832, -58.9281) ccw
  arc A1217 (80.6332, -58.9281) -> (79.1332, -58.9281) centre (79.8832, -58.9281) ccw
  arc A1218 (80.6332, -58.9281) -> (79.1332, -58.9281) centre (79.8832, -58.9281) ccw
  arc A1219 (79.1332, -58.9281) -> (80.6332, -58.9281) centre (79.8832, -58.9281) ccw
  arc A1220 (80.6332, -58.9281) -> (79.1332, -58.9281) centre (79.8832, -58.9281) ccw
  arc A1221 (79.1332, -58.9281) -> (80.6332, -58.9281) centre (79.8832, -58.9281) ccw
  arc A1222 (79.1332, -56.3881) -> (80.6332, -56.3881) centre (79.8832, -56.3881) ccw
  arc A1223 (80.6332, -56.3881) -> (79.1332, -56.3881) centre (79.8832, -56.3881) ccw
  arc A1224 (80.6332, -56.3881) -> (79.1332, -56.3881) centre (79.8832, -56.3881) ccw
  arc A1225 (79.1332, -56.3881) -> (80.6332, -56.3881) centre (79.8832, -56.3881) ccw
  arc A1226 (79.1332, -56.3881) -> (80.6332, -56.3881) centre (79.8832, -56.3881) ccw
  arc A1227 (80.6332, -56.3881) -> (79.1332, -56.3881) centre (79.8832, -56.3881) ccw
  arc A1228 (80.6332, -53.8481) -> (79.1332, -53.8481) centre (79.8832, -53.8481) ccw
  arc A1229 (79.1332, -53.8481) -> (80.6332, -53.8481) centre (79.8832, -53.8481) ccw
  arc A1230 (80.6332, -53.8481) -> (79.1332, -53.8481) centre (79.8832, -53.8481) ccw
  arc A1231 (79.1332, -53.8481) -> (80.6332, -53.8481) centre (79.8832, -53.8481) ccw
  arc A1232 (80.6332, -53.8481) -> (79.1332, -53.8481) centre (79.8832, -53.8481) ccw
  arc A1233 (79.1332, -53.8481) -> (80.6332, -53.8481) centre (79.8832, -53.8481) ccw
  arc A1234 (79.1332, -51.3081) -> (80.6332, -51.3081) centre (79.8832, -51.3081) ccw
  arc A1235 (80.6332, -51.3081) -> (79.1332, -51.3081) centre (79.8832, -51.3081) ccw
  arc A1236 (79.1332, -51.3081) -> (80.6332, -51.3081) centre (79.8832, -51.3081) ccw
  arc A1237 (80.6332, -51.3081) -> (79.1332, -51.3081) centre (79.8832, -51.3081) ccw
  arc A1238 (80.6332, -51.3081) -> (79.1332, -51.3081) centre (79.8832, -51.3081) ccw
  arc A1239 (79.1332, -51.3081) -> (80.6332, -51.3081) centre (79.8832, -51.3081) ccw
  arc A1240 (79.1332, -48.7681) -> (80.6332, -48.7681) centre (79.8832, -48.7681) ccw
  arc A1241 (80.6332, -48.7681) -> (79.1332, -48.7681) centre (79.8832, -48.7681) ccw
  arc A1242 (79.1332, -48.7681) -> (80.6332, -48.7681) centre (79.8832, -48.7681) ccw
  arc A1243 (80.6332, -48.7681) -> (79.1332, -48.7681) centre (79.8832, -48.7681) ccw
  arc A1244 (80.6332, -48.7681) -> (79.1332, -48.7681) centre (79.8832, -48.7681) ccw
  arc A1245 (79.1332, -48.7681) -> (80.6332, -48.7681) centre (79.8832, -48.7681) ccw
  arc A1246 (80.6332, -46.2281) -> (79.1332, -46.2281) centre (79.8832, -46.2281) ccw
  arc A1247 (79.1332, -46.2281) -> (80.6332, -46.2281) centre (79.8832, -46.2281) ccw
  arc A1248 (79.1332, -46.2281) -> (80.6332, -46.2281) centre (79.8832, -46.2281) ccw
  arc A1249 (80.6332, -46.2281) -> (79.1332, -46.2281) centre (79.8832, -46.2281) ccw
  arc A1250 (80.6332, -46.2281) -> (79.1332, -46.2281) centre (79.8832, -46.2281) ccw
  arc A1251 (79.1332, -46.2281) -> (80.6332, -46.2281) centre (79.8832, -46.2281) ccw
  arc A1252 (80.6332, -43.6881) -> (79.1332, -43.6881) centre (79.8832, -43.6881) ccw
  arc A1253 (79.1332, -43.6881) -> (80.6332, -43.6881) centre (79.8832, -43.6881) ccw
  arc A1254 (79.1332, -43.6881) -> (80.6332, -43.6881) centre (79.8832, -43.6881) ccw
  arc A1255 (80.6332, -43.6881) -> (79.1332, -43.6881) centre (79.8832, -43.6881) ccw
  arc A1256 (80.6332, -43.6881) -> (79.1332, -43.6881) centre (79.8832, -43.6881) ccw
  arc A1257 (79.1332, -43.6881) -> (80.6332, -43.6881) centre (79.8832, -43.6881) ccw
  arc A1258 (79.1332, -41.1481) -> (80.6332, -41.1481) centre (79.8832, -41.1481) ccw
  arc A1259 (80.6332, -41.1481) -> (79.1332, -41.1481) centre (79.8832, -41.1481) ccw
  arc A1260 (79.1332, -41.1481) -> (80.6332, -41.1481) centre (79.8832, -41.1481) ccw
  arc A1261 (80.6332, -41.1481) -> (79.1332, -41.1481) centre (79.8832, -41.1481) ccw
  arc A1262 (79.1332, -41.1481) -> (80.6332, -41.1481) centre (79.8832, -41.1481) ccw
  arc A1263 (80.6332, -41.1481) -> (79.1332, -41.1481) centre (79.8832, -41.1481) ccw
  arc A1264 (79.1332, -38.6081) -> (80.6332, -38.6081) centre (79.8832, -38.6081) ccw
  arc A1265 (80.6332, -38.6081) -> (79.1332, -38.6081) centre (79.8832, -38.6081) ccw
  arc A1266 (80.6332, -38.6081) -> (79.1332, -38.6081) centre (79.8832, -38.6081) ccw
  arc A1267 (79.1332, -38.6081) -> (80.6332, -38.6081) centre (79.8832, -38.6081) ccw
  arc A1268 (79.1332, -38.6081) -> (80.6332, -38.6081) centre (79.8832, -38.6081) ccw
  arc A1269 (80.6332, -38.6081) -> (79.1332, -38.6081) centre (79.8832, -38.6081) ccw
  arc A1270 (80.6332, -36.0681) -> (79.1332, -36.0681) centre (79.8832, -36.0681) ccw
  arc A1271 (79.1332, -36.0681) -> (80.6332, -36.0681) centre (79.8832, -36.0681) ccw
  arc A1272 (79.1332, -36.0681) -> (80.6332, -36.0681) centre (79.8832, -36.0681) ccw
  arc A1273 (80.6332, -36.0681) -> (79.1332, -36.0681) centre (79.8832, -36.0681) ccw
  arc A1274 (79.1332, -36.0681) -> (80.6332, -36.0681) centre (79.8832, -36.0681) ccw
  arc A1275 (80.6332, -36.0681) -> (79.1332, -36.0681) centre (79.8832, -36.0681) ccw
  arc A1276 (73.0131, -69.0881) -> (71.5131, -69.0881) centre (72.2631, -69.0881) ccw
  arc A1277 (71.5131, -69.0881) -> (73.0131, -69.0881) centre (72.2631, -69.0881) ccw
  arc A1278 (71.5131, -69.0881) -> (73.0131, -69.0881) centre (72.2631, -69.0881) ccw
  arc A1279 (73.0131, -69.0881) -> (71.5131, -69.0881) centre (72.2631, -69.0881) ccw
  arc A1280 (71.5131, -69.0881) -> (73.0131, -69.0881) centre (72.2631, -69.0881) ccw
  arc A1281 (73.0131, -69.0881) -> (71.5131, -69.0881) centre (72.2631, -69.0881) ccw
  arc A1282 (73.0131, -66.5481) -> (71.5131, -66.5481) centre (72.2631, -66.5481) ccw
  arc A1283 (71.5131, -66.5481) -> (73.0131, -66.5481) centre (72.2631, -66.5481) ccw
  arc A1284 (71.5131, -66.5481) -> (73.0131, -66.5481) centre (72.2631, -66.5481) ccw
  arc A1285 (73.0131, -66.5481) -> (71.5131, -66.5481) centre (72.2631, -66.5481) ccw
  arc A1286 (71.5131, -66.5481) -> (73.0131, -66.5481) centre (72.2631, -66.5481) ccw
  arc A1287 (73.0131, -66.5481) -> (71.5131, -66.5481) centre (72.2631, -66.5481) ccw
  arc A1288 (71.5131, -64.0081) -> (73.0131, -64.0081) centre (72.2631, -64.0081) ccw
  arc A1289 (73.0131, -64.0081) -> (71.5131, -64.0081) centre (72.2631, -64.0081) ccw
  arc A1290 (73.0131, -64.0081) -> (71.5131, -64.0081) centre (72.2631, -64.0081) ccw
  arc A1291 (71.5131, -64.0081) -> (73.0131, -64.0081) centre (72.2631, -64.0081) ccw
  arc A1292 (73.0131, -64.0081) -> (71.5131, -64.0081) centre (72.2631, -64.0081) ccw
  arc A1293 (71.5131, -64.0081) -> (73.0131, -64.0081) centre (72.2631, -64.0081) ccw
  arc A1294 (73.0131, -61.4681) -> (71.5131, -61.4681) centre (72.2631, -61.4681) ccw
  arc A1295 (71.5131, -61.4681) -> (73.0131, -61.4681) centre (72.2631, -61.4681) ccw
  arc A1296 (71.5131, -61.4681) -> (73.0131, -61.4681) centre (72.2631, -61.4681) ccw
  arc A1297 (73.0131, -61.4681) -> (71.5131, -61.4681) centre (72.2631, -61.4681) ccw
  arc A1298 (71.5131, -61.4681) -> (73.0131, -61.4681) centre (72.2631, -61.4681) ccw
  arc A1299 (73.0131, -61.4681) -> (71.5131, -61.4681) centre (72.2631, -61.4681) ccw
  arc A1300 (71.5131, -58.9281) -> (73.0131, -58.9281) centre (72.2631, -58.9281) ccw
  arc A1301 (73.0131, -58.9281) -> (71.5131, -58.9281) centre (72.2631, -58.9281) ccw
  arc A1302 (73.0131, -58.9281) -> (71.5131, -58.9281) centre (72.2631, -58.9281) ccw
  arc A1303 (71.5131, -58.9281) -> (73.0131, -58.9281) centre (72.2631, -58.9281) ccw
  arc A1304 (73.0131, -58.9281) -> (71.5131, -58.9281) centre (72.2631, -58.9281) ccw
  arc A1305 (71.5131, -58.9281) -> (73.0131, -58.9281) centre (72.2631, -58.9281) ccw
  arc A1306 (73.0131, -56.3881) -> (71.5131, -56.3881) centre (72.2631, -56.3881) ccw
  arc A1307 (71.5131, -56.3881) -> (73.0131, -56.3881) centre (72.2631, -56.3881) ccw
  arc A1308 (71.5131, -56.3881) -> (73.0131, -56.3881) centre (72.2631, -56.3881) ccw
  arc A1309 (73.0131, -56.3881) -> (71.5131, -56.3881) centre (72.2631, -56.3881) ccw
  arc A1310 (71.5131, -56.3881) -> (73.0131, -56.3881) centre (72.2631, -56.3881) ccw
  arc A1311 (73.0131, -56.3881) -> (71.5131, -56.3881) centre (72.2631, -56.3881) ccw
  arc A1312 (73.0131, -53.8481) -> (71.5131, -53.8481) centre (72.2631, -53.8481) ccw
  arc A1313 (71.5131, -53.8481) -> (73.0131, -53.8481) centre (72.2631, -53.8481) ccw
  arc A1314 (71.5131, -53.8481) -> (73.0131, -53.8481) centre (72.2631, -53.8481) ccw
  arc A1315 (73.0131, -53.8481) -> (71.5131, -53.8481) centre (72.2631, -53.8481) ccw
  arc A1316 (71.5131, -53.8481) -> (73.0131, -53.8481) centre (72.2631, -53.8481) ccw
  arc A1317 (73.0131, -53.8481) -> (71.5131, -53.8481) centre (72.2631, -53.8481) ccw
  arc A1318 (73.0131, -51.3081) -> (71.5131, -51.3081) centre (72.2631, -51.3081) ccw
  arc A1319 (71.5131, -51.3081) -> (73.0131, -51.3081) centre (72.2631, -51.3081) ccw
  arc A1320 (71.5131, -51.3081) -> (73.0131, -51.3081) centre (72.2631, -51.3081) ccw
  arc A1321 (73.0131, -51.3081) -> (71.5131, -51.3081) centre (72.2631, -51.3081) ccw
  arc A1322 (71.5131, -51.3081) -> (73.0131, -51.3081) centre (72.2631, -51.3081) ccw
  arc A1323 (73.0131, -51.3081) -> (71.5131, -51.3081) centre (72.2631, -51.3081) ccw
  arc A1324 (71.5131, -48.7681) -> (73.0131, -48.7681) centre (72.2631, -48.7681) ccw
  arc A1325 (73.0131, -48.7681) -> (71.5131, -48.7681) centre (72.2631, -48.7681) ccw
  arc A1326 (73.0131, -48.7681) -> (71.5131, -48.7681) centre (72.2631, -48.7681) ccw
  arc A1327 (71.5131, -48.7681) -> (73.0131, -48.7681) centre (72.2631, -48.7681) ccw
  arc A1328 (73.0131, -48.7681) -> (71.5131, -48.7681) centre (72.2631, -48.7681) ccw
  arc A1329 (71.5131, -48.7681) -> (73.0131, -48.7681) centre (72.2631, -48.7681) ccw
  arc A1330 (71.5131, -46.2281) -> (73.0131, -46.2281) centre (72.2631, -46.2281) ccw
  arc A1331 (73.0131, -46.2281) -> (71.5131, -46.2281) centre (72.2631, -46.2281) ccw
  arc A1332 (73.0131, -46.2281) -> (71.5131, -46.2281) centre (72.2631, -46.2281) ccw
  arc A1333 (71.5131, -46.2281) -> (73.0131, -46.2281) centre (72.2631, -46.2281) ccw
  arc A1334 (73.0131, -46.2281) -> (71.5131, -46.2281) centre (72.2631, -46.2281) ccw
  arc A1335 (71.5131, -46.2281) -> (73.0131, -46.2281) centre (72.2631, -46.2281) ccw
  arc A1336 (71.5131, -43.6881) -> (73.0131, -43.6881) centre (72.2631, -43.6881) ccw
  arc A1337 (73.0131, -43.6881) -> (71.5131, -43.6881) centre (72.2631, -43.6881) ccw
  arc A1338 (71.5131, -43.6881) -> (73.0131, -43.6881) centre (72.2631, -43.6881) ccw
  arc A1339 (73.0131, -43.6881) -> (71.5131, -43.6881) centre (72.2631, -43.6881) ccw
  arc A1340 (71.5131, -43.6881) -> (73.0131, -43.6881) centre (72.2631, -43.6881) ccw
  arc A1341 (73.0131, -43.6881) -> (71.5131, -43.6881) centre (72.2631, -43.6881) ccw
  arc A1342 (73.0131, -41.1481) -> (71.5131, -41.1481) centre (72.2631, -41.1481) ccw
  arc A1343 (71.5131, -41.1481) -> (73.0131, -41.1481) centre (72.2631, -41.1481) ccw
  arc A1344 (71.5131, -41.1481) -> (73.0131, -41.1481) centre (72.2631, -41.1481) ccw
  arc A1345 (73.0131, -41.1481) -> (71.5131, -41.1481) centre (72.2631, -41.1481) ccw
  arc A1346 (71.5131, -41.1481) -> (73.0131, -41.1481) centre (72.2631, -41.1481) ccw
  arc A1347 (73.0131, -41.1481) -> (71.5131, -41.1481) centre (72.2631, -41.1481) ccw
  arc A1348 (71.5131, -38.6081) -> (73.0131, -38.6081) centre (72.2631, -38.6081) ccw
  arc A1349 (73.0131, -38.6081) -> (71.5131, -38.6081) centre (72.2631, -38.6081) ccw
  arc A1350 (73.0131, -38.6081) -> (71.5131, -38.6081) centre (72.2631, -38.6081) ccw
  arc A1351 (71.5131, -38.6081) -> (73.0131, -38.6081) centre (72.2631, -38.6081) ccw
  arc A1352 (73.0131, -38.6081) -> (71.5131, -38.6081) centre (72.2631, -38.6081) ccw
  arc A1353 (71.5131, -38.6081) -> (73.0131, -38.6081) centre (72.2631, -38.6081) ccw
  line L244 (71.5131, -35.3181) -> (73.0131, -35.3181)
  line L245 (71.5131, -36.8181) -> (71.5131, -35.3181)
  line L246 (73.0131, -35.3181) -> (73.0131, -36.8181)
  line L247 (73.0131, -36.8181) -> (71.5131, -36.8181)
  line L248 (73.0131, -36.8181) -> (71.5131, -36.8181)
  line L249 (73.0131, -35.3181) -> (73.0131, -36.8181)
  line L250 (71.5131, -36.8181) -> (71.5131, -35.3181)
  line L251 (71.5131, -35.3181) -> (73.0131, -35.3181)
  line L252 (73.0131, -35.3181) -> (73.0131, -36.8181)
  line L253 (71.5131, -35.3181) -> (73.0131, -35.3181)
  line L254 (71.5131, -36.8181) -> (71.5131, -35.3181)
  line L255 (73.0131, -36.8181) -> (71.5131, -36.8181)
  arc A1354 (45.5811, -97.0282) -> (44.0811, -97.0282) centre (44.8311, -97.0282) ccw
  arc A1355 (44.0811, -97.0282) -> (45.5811, -97.0282) centre (44.8311, -97.0282) ccw
  arc A1356 (44.0811, -97.0282) -> (45.5811, -97.0282) centre (44.8311, -97.0282) ccw
  arc A1357 (45.5811, -97.0282) -> (44.0811, -97.0282) centre (44.8311, -97.0282) ccw
  arc A1358 (44.0811, -97.0282) -> (45.5811, -97.0282) centre (44.8311, -97.0282) ccw
  arc A1359 (45.5811, -97.0282) -> (44.0811, -97.0282) centre (44.8311, -97.0282) ccw
  arc A1360 (48.1211, -97.0282) -> (46.6211, -97.0282) centre (47.3711, -97.0282) ccw
  arc A1361 (46.6211, -97.0282) -> (48.1211, -97.0282) centre (47.3711, -97.0282) ccw
  arc A1362 (48.1211, -97.0282) -> (46.6211, -97.0282) centre (47.3711, -97.0282) ccw
  arc A1363 (46.6211, -97.0282) -> (48.1211, -97.0282) centre (47.3711, -97.0282) ccw
  arc A1364 (48.1211, -97.0282) -> (46.6211, -97.0282) centre (47.3711, -97.0282) ccw
  arc A1365 (46.6211, -97.0282) -> (48.1211, -97.0282) centre (47.3711, -97.0282) ccw
  arc A1366 (49.1611, -97.0282) -> (50.6611, -97.0282) centre (49.9111, -97.0282) ccw
  arc A1367 (50.6611, -97.0282) -> (49.1611, -97.0282) centre (49.9111, -97.0282) ccw
  arc A1368 (50.6611, -97.0282) -> (49.1611, -97.0282) centre (49.9111, -97.0282) ccw
  arc A1369 (49.1611, -97.0282) -> (50.6611, -97.0282) centre (49.9111, -97.0282) ccw
  arc A1370 (49.1611, -97.0282) -> (50.6611, -97.0282) centre (49.9111, -97.0282) ccw
  arc A1371 (50.6611, -97.0282) -> (49.1611, -97.0282) centre (49.9111, -97.0282) ccw
  arc A1372 (53.2011, -97.0282) -> (51.7011, -97.0282) centre (52.4511, -97.0282) ccw
  arc A1373 (51.7011, -97.0282) -> (53.2011, -97.0282) centre (52.4511, -97.0282) ccw
  arc A1374 (53.2011, -97.0282) -> (51.7011, -97.0282) centre (52.4511, -97.0282) ccw
  arc A1375 (51.7011, -97.0282) -> (53.2011, -97.0282) centre (52.4511, -97.0282) ccw
  arc A1376 (51.7011, -97.0282) -> (53.2011, -97.0282) centre (52.4511, -97.0282) ccw
  arc A1377 (53.2011, -97.0282) -> (51.7011, -97.0282) centre (52.4511, -97.0282) ccw
  arc A1378 (54.2411, -97.0282) -> (55.7411, -97.0282) centre (54.9911, -97.0282) ccw
  arc A1379 (55.7411, -97.0282) -> (54.2411, -97.0282) centre (54.9911, -97.0282) ccw
  arc A1380 (54.2411, -97.0282) -> (55.7411, -97.0282) centre (54.9911, -97.0282) ccw
  arc A1381 (55.7411, -97.0282) -> (54.2411, -97.0282) centre (54.9911, -97.0282) ccw
  arc A1382 (54.2411, -97.0282) -> (55.7411, -97.0282) centre (54.9911, -97.0282) ccw
  arc A1383 (55.7411, -97.0282) -> (54.2411, -97.0282) centre (54.9911, -97.0282) ccw
  arc A1384 (56.7811, -97.0282) -> (58.2811, -97.0282) centre (57.5311, -97.0282) ccw
  arc A1385 (58.2811, -97.0282) -> (56.7811, -97.0282) centre (57.5311, -97.0282) ccw
  arc A1386 (58.2811, -97.0282) -> (56.7811, -97.0282) centre (57.5311, -97.0282) ccw
  arc A1387 (56.7811, -97.0282) -> (58.2811, -97.0282) centre (57.5311, -97.0282) ccw
  arc A1388 (56.7811, -97.0282) -> (58.2811, -97.0282) centre (57.5311, -97.0282) ccw
  arc A1389 (58.2811, -97.0282) -> (56.7811, -97.0282) centre (57.5311, -97.0282) ccw
  arc A1390 (60.8211, -97.0282) -> (59.3211, -97.0282) centre (60.0711, -97.0282) ccw
  arc A1391 (59.3211, -97.0282) -> (60.8211, -97.0282) centre (60.0711, -97.0282) ccw
  arc A1392 (60.8211, -97.0282) -> (59.3211, -97.0282) centre (60.0711, -97.0282) ccw
  arc A1393 (59.3211, -97.0282) -> (60.8211, -97.0282) centre (60.0711, -97.0282) ccw
  arc A1394 (60.8211, -97.0282) -> (59.3211, -97.0282) centre (60.0711, -97.0282) ccw
  arc A1395 (59.3211, -97.0282) -> (60.8211, -97.0282) centre (60.0711, -97.0282) ccw
  arc A1396 (63.3611, -97.0282) -> (61.8611, -97.0282) centre (62.6111, -97.0282) ccw
  arc A1397 (61.8611, -97.0282) -> (63.3611, -97.0282) centre (62.6111, -97.0282) ccw
  arc A1398 (61.8611, -97.0282) -> (63.3611, -97.0282) centre (62.6111, -97.0282) ccw
  arc A1399 (63.3611, -97.0282) -> (61.8611, -97.0282) centre (62.6111, -97.0282) ccw
  arc A1400 (63.3611, -97.0282) -> (61.8611, -97.0282) centre (62.6111, -97.0282) ccw
  arc A1401 (61.8611, -97.0282) -> (63.3611, -97.0282) centre (62.6111, -97.0282) ccw
  arc A1402 (64.4011, -97.0282) -> (65.9011, -97.0282) centre (65.1511, -97.0282) ccw
  arc A1403 (65.9011, -97.0282) -> (64.4011, -97.0282) centre (65.1511, -97.0282) ccw
  arc A1404 (65.9011, -97.0282) -> (64.4011, -97.0282) centre (65.1511, -97.0282) ccw
  arc A1405 (64.4011, -97.0282) -> (65.9011, -97.0282) centre (65.1511, -97.0282) ccw
  arc A1406 (64.4011, -97.0282) -> (65.9011, -97.0282) centre (65.1511, -97.0282) ccw
  arc A1407 (65.9011, -97.0282) -> (64.4011, -97.0282) centre (65.1511, -97.0282) ccw
  arc A1408 (68.4411, -97.0282) -> (66.9411, -97.0282) centre (67.6911, -97.0282) ccw
  arc A1409 (66.9411, -97.0282) -> (68.4411, -97.0282) centre (67.6911, -97.0282) ccw
  arc A1410 (66.9411, -97.0282) -> (68.4411, -97.0282) centre (67.6911, -97.0282) ccw
  arc A1411 (68.4411, -97.0282) -> (66.9411, -97.0282) centre (67.6911, -97.0282) ccw
  arc A1412 (68.4411, -97.0282) -> (66.9411, -97.0282) centre (67.6911, -97.0282) ccw
  arc A1413 (66.9411, -97.0282) -> (68.4411, -97.0282) centre (67.6911, -97.0282) ccw
  arc A1414 (69.4811, -97.0282) -> (70.9811, -97.0282) centre (70.2311, -97.0282) ccw
  arc A1415 (70.9811, -97.0282) -> (69.4811, -97.0282) centre (70.2311, -97.0282) ccw
  arc A1416 (70.9811, -97.0282) -> (69.4811, -97.0282) centre (70.2311, -97.0282) ccw
  arc A1417 (69.4811, -97.0282) -> (70.9811, -97.0282) centre (70.2311, -97.0282) ccw
  arc A1418 (69.4811, -97.0282) -> (70.9811, -97.0282) centre (70.2311, -97.0282) ccw
  arc A1419 (70.9811, -97.0282) -> (69.4811, -97.0282) centre (70.2311, -97.0282) ccw
  arc A1420 (72.0211, -97.0282) -> (73.5211, -97.0282) centre (72.7711, -97.0282) ccw
  arc A1421 (73.5211, -97.0282) -> (72.0211, -97.0282) centre (72.7711, -97.0282) ccw
  arc A1422 (73.5211, -97.0282) -> (72.0211, -97.0282) centre (72.7711, -97.0282) ccw
  arc A1423 (72.0211, -97.0282) -> (73.5211, -97.0282) centre (72.7711, -97.0282) ccw
  arc A1424 (73.5211, -97.0282) -> (72.0211, -97.0282) centre (72.7711, -97.0282) ccw
  arc A1425 (72.0211, -97.0282) -> (73.5211, -97.0282) centre (72.7711, -97.0282) ccw
  arc A1426 (76.0612, -97.0282) -> (74.5612, -97.0282) centre (75.3112, -97.0282) ccw
  arc A1427 (74.5612, -97.0282) -> (76.0612, -97.0282) centre (75.3112, -97.0282) ccw
  arc A1428 (74.5612, -97.0282) -> (76.0612, -97.0282) centre (75.3112, -97.0282) ccw
  arc A1429 (76.0612, -97.0282) -> (74.5612, -97.0282) centre (75.3112, -97.0282) ccw
  arc A1430 (74.5612, -97.0282) -> (76.0612, -97.0282) centre (75.3112, -97.0282) ccw
  arc A1431 (76.0612, -97.0282) -> (74.5612, -97.0282) centre (75.3112, -97.0282) ccw
  arc A1432 (78.6012, -97.0282) -> (77.1012, -97.0282) centre (77.8512, -97.0282) ccw
  arc A1433 (77.1012, -97.0282) -> (78.6012, -97.0282) centre (77.8512, -97.0282) ccw
  arc A1434 (78.6012, -97.0282) -> (77.1012, -97.0282) centre (77.8512, -97.0282) ccw